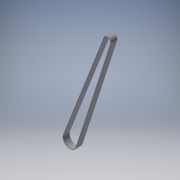
# Autodesk Inventor part: Belt
Saved by Autodesk Inventor 2017 (Build 210142000, 142)
## iProperties
Created: 2020-02-22
Part Number: Belt
Material: Generic
Document SubType Name: Modeling
Designer: S346553810
Density: 1 g/cm^3
Appearance: Default
Author: S346553810
Autodesk Inventor part; units mm, degrees
ref_plane "YZ Plane" through (0, 0, 0) normal (1, 0, 0) x (0, 1, 0)
ref_plane "XZ Plane" through (0, 0, 0) normal (0, 1, 0) x (-1, 0, 0)
ref_plane "XY Plane" through (0, 0, 0) normal (0, 0, 1) x (1, 0, 0)
ref_plane "Work Plane1" through (0, 0, 0) normal (0, 0, 1) x (1, 0, 0)
sketch "Sketch1" plane through (0, 0, 0) normal (0, 0, 1) x (1, 0, 0)
  arc A0 (7.5768, -31.9111) -> (11.0096, -30.8953) centre (0, 0) ccw construction
  arc A1 (2.7361, -32.684) -> (6.282, -32.1911) centre (0, 0) ccw construction
  arc A2 (-2.1658, -32.7267) -> (1.414, -32.7678) centre (0, 0) ccw construction
  arc A3 (12.2483, -30.4254) -> (15.4914, -28.9093) centre (0, 0) ccw construction
  arc A4 (16.6462, -28.2601) -> (19.627, -26.2775) centre (0, 0) ccw construction
  circle A5 centre (0, 0) radius 37.1131 construction
  circle A6 centre (0, 0) radius 32.4639 construction
  arc A7 (-32.3268, 5.5412) -> (28.3967, -16.412) centre (0, 0) ccw
  circle A8 centre (185.9759, 522.491) radius 15.875 construction
  circle A9 centre (185.9759, 522.491) radius 6.35 construction
  arc A10 (198.6184, 512.8898) -> (171.693, 529.4203) centre (185.9759, 522.491) ccw construction
  arc A11 (200.9863, 517.3234) -> (171.693, 529.4203) centre (185.9759, 522.491) ccw
  line L0 (200.9863, 517.3234) -> (28.3967, -16.412)
  line L1 (-32.3268, 5.5412) -> (171.693, 529.4203)
  arc A12 (203.396, 516.52) -> (169.3619, 530.4337) centre (185.9759, 522.491) ccw
  line L2 (203.396, 516.52) -> (30.7322, -17.445)
  arc A13 (-34.7852, 6.228) -> (30.7322, -17.445) centre (0, 0) ccw
  line L3 (-34.7852, 6.228) -> (169.3619, 530.4337)
  dimension "d0" = 2.54
  constraints: 16 point on circle, 8 end point, 6 centre point, 2 concentric, 4 other
  measures "d0" distance between parallel lines of L1 L3
extrude "Extrusion1" add sketch "Sketch1" along normal up to surface (30.8991 mm away)
body "Solid1"
